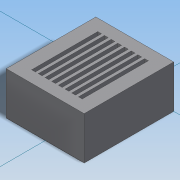
# Autodesk Inventor part: ESC HK-200A
Saved by Autodesk Inventor 2014 SP2 (Build 180246200, 246)
## iProperties
Created: 2014-05-19
Part Number: ESC HK-200A
Material: Generic
Document SubType Name: Modeling
Designer: dliu
Density: 1 g/cm^3
Appearance: Default
Author: dliu
Autodesk Inventor part; units mm, degrees
ref_plane "YZ Plane" through (0, 0, 0) normal (1, 0, 0) x (0, 1, 0)
ref_plane "XZ Plane" through (0, 0, 0) normal (0, 1, 0) x (-1, 0, 0)
ref_plane "XY Plane" through (0, 0, 0) normal (0, 0, 1) x (1, 0, 0)
sketch "Sketch1" plane through (0, 0, 0) normal (0, 0, 1) x (1, 0, 0)
  line L0 (-20, 11) -> (20, 11)
  line L1 (20, 11) -> (20, -11)
  line L2 (20, -11) -> (-20, -11)
  line L3 (-20, -11) -> (-20, 11)
  line L4 (-20, 11) -> (20, -11) construction
  line L5 (20, 11) -> (-20, -11) construction
  point P0 (0, 0)
  dimension "d0" = 40
  dimension "d1" = 22
  constraints: 12 end point, 2 midpoint, 2 parallel, 1 horizontal, 1 perpendicular
  measures "d0" distance of L1.end L2.end
  measures "d1" distance of L0.end L1.end
extrude "Extrusion1" add sketch "Sketch1" along normal blind 46
sketch "Sketch2" plane through (-20, 11, 0) normal (0, 1, 0) x (1, 0, 0)
  line L0 (0, 0) -> (40, 0) construction
  line L1 (0, 0) -> (0, -46) construction
  line L2 (40, -46) -> (0, -46) construction
  line L3 (40, 0) -> (40, -46) construction
  line L4 (0, 0) -> (40, -46) construction
  line L5 (0, -46) -> (40, 0) construction
  line L6 (7, -6) -> (33, -6)
  line L7 (33, -6) -> (33, -40)
  line L8 (33, -40) -> (7, -40)
  line L9 (7, -40) -> (7, -6)
  line L10 (7, -6) -> (33, -40) construction
  line L11 (33, -6) -> (7, -40) construction
  point P0 (20, 0)
  point P1 (20, -23)
  dimension "d4" = 26
  dimension "d5" = 34
  constraints: 16 end point, 3 midpoint, 2 parallel, 1 horizontal, 1 perpendicular
  measures "d4" distance of L7.end L8.end
  measures "d5" distance of L6.end L7.end
extrude "Heatsink Cut" cut sketch "Sketch2" against normal blind 5
sketch "Sketch3" plane through (-20, 11, 0) normal (0, 1, 0) x (1, 0, 0)
  line L0 (7, -6) -> (33, -6) projected
  line L1 (7, -40) -> (7, -6) projected
  line L2 (33, -40) -> (7, -40) projected
  line L3 (33, -6) -> (33, -40) projected
  line L4 (8.9375, -6) -> (10.4375, -6)
  line L5 (10.4375, -6) -> (10.4375, -40)
  line L6 (10.4375, -40) -> (8.9375, -40)
  line L7 (8.9375, -40) -> (8.9375, -6)
  point P0 (20, 0)
  dimension "d8" = 1.5
  dimension "d9" = 26
  dimension "d10" = 1.9375
  constraints: 8 end point, 2 parallel, 2 point on line, 1 horizontal, 1 perpendicular
  measures "d8" distance between parallel lines of L5 L7
  measures "d9" distance between parallel lines of L3 L1
  measures "d10" distance between parallel lines of L7 L1
extrude "Heatsink Fin" add sketch "Sketch3" against normal up to next contours L0 L5 L2 L7
pattern_linear "Rectangular Pattern1" count 7 spacing 3.4375 along (1, 0, 0) of "Heatsink Fin"
fillet "Fillet4" radius 0.635 14 edges at (-11.0625, 11, 23) (-9.5625, 11, 23) (-7.625, 11, 23) (-6.125, 11, 23) (-4.1875, 11, 23) (-2.6875, 11, 23) (-0.75, 11, 23) (0.75, 11, 23) (2.6875, 11, 23) (4.1875, 11, 23) (6.125, 11, 23) (7.625, 11, 23) (9.5625, 11, 23) (11.0625, 11, 23)
sketch "Sketch4" plane through (0, 0, 46) normal (0, 0, 1) x (1, 0, 0)
  line L0 (20, 11) -> (-20, 11) projected
  line L1 (-20, 11) -> (-20, -11) projected
  line L2 (-20, -11) -> (20, -11) projected
  line L3 (20, -11) -> (20, 11) projected
  line L4 (-20, 2.5) -> (-9.2101, 2.5) construction
  line L5 (19.9799, 2.5) -> (19.9799, -15.5)
  line L6 (19.9799, -15.5) -> (-20, -15.5)
  line L7 (-20, -15.5) -> (-9.2101, 2.5)
  line L8 (19.9799, -15.5) -> (17.1371, -11)
  line L9 (17.1371, -11) -> (9.1899, 2.5)
  line L10 (9.1899, 2.5) -> (19.9799, 2.5) construction
  line L11 (-9.2101, 2.5) -> (9.1899, 2.5)
  point P0 (0, 0)
  dimension "d16" = 4.5
  dimension "d17" = 18
  dimension "d23" = 18.4
  constraints: 16 end point, 3 horizontal, 3 parallel, 3 perpendicular, 2 point on line, 1 collinear
  measures "d16" distance between parallel lines of L6 L2
  measures "d17" distance between parallel lines of L6 L4
  measures "d23" distance of L4.end L9.end
extrude "Wires and Caps Bundle" add sketch "Sketch4" along normal blind 26 contours L7 L11 L9 L2 | L2 L8 L6 L7
sketch "Sketch5" plane through (0, 0, 0) normal (0, 0, -1) x (-1, 0, 0)
  line L0 (-15, 4.2) -> (15, 4.2)
  line L1 (15, 4.2) -> (15, -5.8)
  line L2 (15, -5.8) -> (-15, -5.8)
  line L3 (-15, -5.8) -> (-15, 4.2)
  line L4 (20, 11) -> (-20, 11) projected
  line L5 (-20, 11) -> (-20, -11) construction
  line L6 (-15, -0.8) -> (-20, -0.8) construction
  line L7 (15, -0.8) -> (20, -0.8) construction
  line L8 (20, -11) -> (20, 11) construction
  point P0 (0, 0)
  dimension "d28" = 30
  dimension "d29" = 10
  dimension "d30" = 6.8
  constraints: 12 end point, 3 equal length, 2 midpoint, 2 perpendicular, 2 point on line, 1 collinear, 1 horizontal
  measures "d28" distance of L1.end L2.end
  measures "d29" distance of L0.end L1.end
  measures "d30" distance between parallel lines of L0 L4
extrude "Output Wires Bundle" add sketch "Sketch5" along normal blind 18.3
chamfer "Chamfer1" distance 4.5 distance2 4.5 1 edges at (-0.0101, -15.5, 46) measured on face at (-0.0101, -15.5, 46.5)
fillet "Fillet1" radius 12.7 2 edges at (9.1899, 2.5, 59) (-9.2101, 2.5, 59)
fillet "Fillet2" radius 2 2 edges at (-20, -15.5, 61.25) (19.9799, -15.5, 61.25)
fillet "Fillet3" radius 2.54 11 edges at (-20, 0, 46) (0, 11, 46) (-20, 11, 23) (0, 11, 0) (20, 11, 23) (0, -11, 0) (-20, -11, 23) (20, -11, 23) (20, 0, 46) (20, 0, 0) (-20, 0, 0)
fillet "Fillet5" radius 6.35 4 edges at (-15, 4.2, -9.15) (-15, -5.8, -9.15) (15, 4.2, -9.15) (15, -5.8, -9.15)
equation "\"d10\" = -0.875 * d8 + 0.125 * d9"
body "Solid1"
